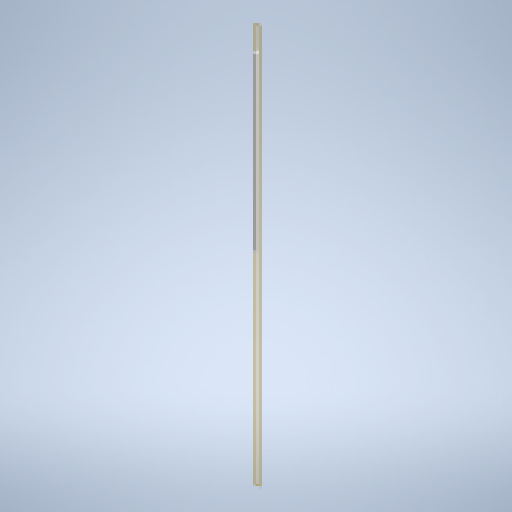
# Autodesk Inventor part: grooves
Saved by Autodesk Inventor 2024 (Build 280153000, 153)
## iProperties
Created: 2024-04-16
Part Number: grooves
Material: Generic
Document SubType Name: Modeling
Designer: teeta
Density: 1 g/cm^3
Appearance: Default
Author: teeta
Autodesk Inventor part; units mm, degrees
ref_plane "YZ Plane" through (0, 0, 0) normal (1, 0, 0) x (0, 1, 0)
ref_plane "XZ Plane" through (0, 0, 0) normal (0, 1, 0) x (-1, 0, 0)
ref_plane "XY Plane" through (0, 0, 0) normal (0, 0, 1) x (1, 0, 0)
ref_plane "Work Plane1" through (0, 0, 0) normal (0, 0, 1) x (1, 0, 0)
sketch "Sketch1" plane through (0, 0, 0) normal (0, 0, 1) x (1, 0, 0)
  line L0 (0, 1159.0752) -> (-10, 1159.0752)
  line L1 (-10, 1159.0752) -> (-10, 615.0291)
  line L2 (-10, 615.0291) -> (0, 615.0291)
  line L3 (0, 615.0291) -> (0, 1159.0752)
  line L4 (-12.7, 1177.775) -> (0, 1177.775) projected
  point P0 (0, 0)
  dimension "d2" = 10
  dimension "d3" = 18.6998
  dimension "d4" = 544.0461
  constraints: 8 end point, 2 parallel, 1 horizontal, 1 perpendicular
  measures "d2" distance between parallel lines of L1 L3
  measures "d3" distance between parallel lines of L4 L0
  measures "d4" distance of L2.end L0.start
extrude "Extrusion1" add sketch "Sketch1" along normal blind 10
body "Solid1"
